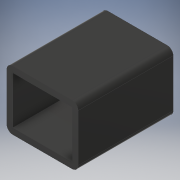
# Autodesk Inventor part: slotcar_adapter
Saved by Autodesk Inventor 2019.4 (Build 234330000, 330)
## iProperties
Created: 2020-09-27
Part Number: slotcar_adapter
Material: Generic
Document SubType Name: Modeling
Designer: deanv
Density: 1 g/cm^3
Appearance: Smooth - Black
Author: deanv
Autodesk Inventor part; units mm, degrees
ref_plane "YZ Plane" through (0, 0, 0) normal (1, 0, 0) x (0, 1, 0)
ref_plane "XZ Plane" through (0, 0, 0) normal (0, 1, 0) x (-1, 0, 0)
ref_plane "XY Plane" through (0, 0, 0) normal (0, 0, 1) x (1, 0, 0)
sketch "Sketch1" plane through (0, 0, 0) normal (0, 0, 1) x (1, 0, 0)
  line L0 (-10, -10) -> (10, -10) construction
  line L1 (10, -10) -> (10, 10) construction
  line L2 (10, 10) -> (-10, 10) construction
  line L3 (-10, 10) -> (-10, -10) construction
  line L4 (-10, -10) -> (10, 10) construction
  line L5 (10, -10) -> (-10, 10) construction
  line L6 (10, -7.5) -> (-10, -7.5) construction
  line L7 (-10, -7.5) -> (-10, 7.5) construction
  line L8 (-10, 7.5) -> (10, 7.5) construction
  line L9 (10, 7.5) -> (10, -7.5) construction
  line L10 (10, -7.5) -> (-10, 7.5) construction
  line L11 (-10, -7.5) -> (10, 7.5) construction
  line L12 (12.5, -10) -> (-12.5, -10)
  line L13 (-12.5, -10) -> (-12.5, 10)
  line L14 (-12.5, 10) -> (12.5, 10)
  line L15 (12.5, 10) -> (12.5, -10)
  line L16 (12.5, -10) -> (-12.5, 10) construction
  line L17 (-12.5, -10) -> (12.5, 10) construction
  line L18 (15, -12.5) -> (-15, -12.5)
  line L19 (-15, -12.5) -> (-15, 12.5)
  line L20 (-15, 12.5) -> (15, 12.5)
  line L21 (15, 12.5) -> (15, -12.5)
  line L22 (15, -12.5) -> (-15, 12.5) construction
  line L23 (-15, -12.5) -> (15, 12.5) construction
  point P0 (0, 0)
  dimension "d0" = 20
  dimension "d1" = 20
  dimension "d2" = 20
  dimension "d3" = 15
  dimension "d4" = 25
  dimension "d5" = 20
  dimension "d6" = 30
  dimension "d7" = 25
  constraints: 48 end point, 8 midpoint, 8 parallel, 4 coincident, 4 horizontal, 4 perpendicular
  measures "d0" distance of L2.end L1.end
  measures "d1" distance of L1.end L0.end
  measures "d2" distance of L7.end L8.end
  measures "d3" distance of L6.end L7.end
  measures "d4" distance of L13.end L14.end
  measures "d5" distance of L12.end L13.end
  measures "d6" distance of L19.end L20.end
  measures "d7" distance of L18.end L19.end
extrude "Extrusion1" add sketch "Sketch1" along normal blind 7.5 contours L12 L13 L14 L15
extrude "Extrusion2" add sketch "Sketch1" along normal blind 40
hole "Hole1" at (-10, 7.5, 0) at (10, 7.5, 0) at (10, -7.5, 0) at (-10, -7.5, 0) direction (0, 0, 1) diameter 2.5 end through all both
fillet "Fillet1" radius 2.5 4 edges at (15, 12.5, 20) (-15, 12.5, 20) (15, -12.5, 20) (-15, -12.5, 20)
body "Solid1"
